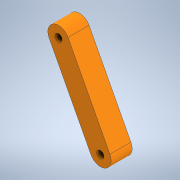
# Autodesk Inventor part: FIRST ARM
Saved by Autodesk Inventor 2021 (Build 250183000, 183)
## iProperties
Created: 2021-07-24
Part Number: FIRST ARM
Material: Generic
Document SubType Name: Modeling
Designer: aksha
Density: 1 g/cm^3
Appearance: Default
Author: aksha
Autodesk Inventor part; units mm, degrees
ref_plane "YZ Plane" through (0, 0, 0) normal (1, 0, 0) x (0, 1, 0)
ref_plane "XZ Plane" through (0, 0, 0) normal (0, 1, 0) x (-1, 0, 0)
ref_plane "XY Plane" through (0, 0, 0) normal (0, 0, 1) x (1, 0, 0)
sketch "Sketch1" plane through (0, 0, 0) normal (0, 0, 1) x (1, 0, 0)
  arc A0 (66.4929, 34.6943) -> (-66.4929, -34.6943) centre (0, 0) ccw
  circle A1 centre (0, 0) radius 25
  arc A2 (226.7447, -596.6943) -> (359.7304, -527.3057) centre (293.2376, -562) ccw
  circle A3 centre (293.2376, -562) radius 25
  line L0 (-66.4929, -34.6943) -> (226.7447, -596.6943)
  line L1 (66.4929, 34.6943) -> (359.7304, -527.3057)
  dimension "d0" = 150
  dimension "d1" = 50
  dimension "d2" = 150
  dimension "d3" = 50
  dimension "d4" = 562
  constraints: 4 centre point, 4 end point, 4 point on circle, 3 coincident, 3 tangent, 1 parallel
  measures "d0" diameter of A0
  measures "d1" diameter of A1
  measures "d2" diameter of A2
  measures "d3" diameter of A3
  measures "d4" vertical distance of A2.centre point (0, 0)
extrude "Extrusion1" add sketch "Sketch1" along normal blind 147
body "Solid1"
